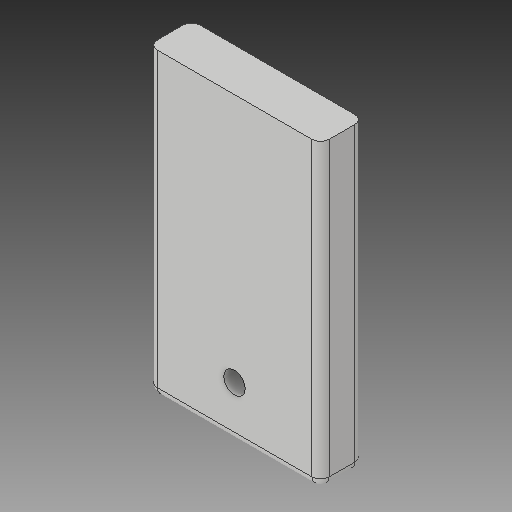
# Autodesk Inventor part: HeadLeverAssemblyAttacher
Saved by Autodesk Inventor 2018 (Build 220112000, 112)
## iProperties
Created: 2018-05-20
Part Number: HeadLeverAssemblyAttacher
Material: Generic
Document SubType Name: Modeling
Designer: reide
Density: 1 g/cm^3
Appearance: Default
Author: reide
Autodesk Inventor part; units mm, degrees
ref_plane "YZ Plane" through (0, 0, 0) normal (1, 0, 0) x (0, 1, 0)
ref_plane "XZ Plane" through (0, 0, 0) normal (0, 1, 0) x (-1, 0, 0)
sketch "Sketch1" plane through (0, 0, 0) normal (0, 0, 1) x (1, 0, 0)
  circle A0 centre (-10, -29) radius 1.25 projected
  line L0 (-20, 0) -> (0, 0) projected
  line L1 (-20, 0) -> (-20, -35) projected
  line L2 (0, -35) -> (-20, -35) projected
  line L3 (0, 0) -> (0, -35) projected
ref_plane "Work Plane1" through (-20, -35, -5) normal (0, 0, -1) x (0, 1, 0)
extrude "Extrusion1" add sketch "Sketch1" against normal up to surface (5 mm away)
fillet "Fillet1" radius 1 4 edges at (-20, -17.5, 0) (-20, -17.5, -5) (0, -17.5, 0) (0, -17.5, -5)
fillet "Fillet2" radius 1 8 edges at (-0.2929, -35, -0.2929) (0, -35, -2.5) (-0.2929, -35, -4.7071) (-10, -35, -5) (-19.7071, -35, -4.7071) (-20, -35, -2.5) (-19.7071, -35, -0.2929) (-10, -35, 0)
body "Solid1"
